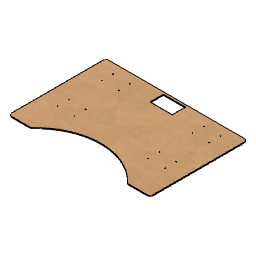
Support_1 (Autodesk Fusion 360 design; units mm, degrees)
Autodesk Fusion 360 part; units mm, degrees
sketch "Esquisse1" plane through (0, 0, 0) normal (0, 1, 0) x (1, 0, 0)
  line L0 (-305, 225) -> (305, 225)
  line L1 (325, 205) -> (325, -205)
  line L2 (305, -225) -> (223.8346, -225)
  line L3 (-325, -205) -> (-325, 205)
  line L4 (-325, 225) -> (325, -225) construction
  line L5 (325, 225) -> (-325, -225) construction
  arc A0 (209.2489, -218.6842) -> (-209.2489, -218.6842) centre (0, -415) ccw
  line L6 (-367.4671, -125) -> (350, -125) construction
  line L7 (-305, -225) -> (-223.8346, -225)
  line L8 (215, -225) -> (325, -225)
  arc A1 (209.2489, -218.6842) -> (223.8346, -225) centre (223.8346, -205) ccw
  arc A2 (305, -225) -> (325, -205) centre (305, -205) ccw
  arc A3 (325, 205) -> (305, 225) centre (305, 205) ccw
  arc A4 (-305, 225) -> (-325, 205) centre (-305, 205) ccw
  arc A5 (-325, -205) -> (-305, -225) centre (-305, -205) ccw
  arc A6 (-223.8346, -225) -> (-209.2489, -218.6842) centre (-223.8346, -205) ccw
  point P0 (-215, -225)
  dimension "d12" = 650
  dimension "d13" = 450
  dimension "d14" = 110
  dimension "d15" = 110
  dimension "d16" = 100
  dimension "d20" = 190
  dimension "d21" = 20
  constraint horizontal L0
  constraint perpendicular L0 L1
  constraint parallel L0 L2
  constraint parallel L1 L3
  constraint coincident L4 origin
  constraint coincident L5 origin
  constraint coincident L2 P0
  constraint perpendicular L1 L6
  constraint perpendicular L1 L8
  constraint tangent A0 A1
  constraint tangent L2 A1
  constraint coincident L4.end L2
  constraint coincident L4.end L1
  constraint tangent L2 A2
  constraint tangent L1 A2
  constraint equal A1 A2
  constraint coincident L5.start L0
  constraint coincident L5.start L1
  constraint tangent L0 A3
  constraint tangent L1 A3
  constraint equal A1 A3
  constraint coincident L4.start L0
  constraint coincident L4.start L3
  constraint tangent L0 A4
  constraint tangent L3 A4
  constraint equal A1 A4
  constraint coincident L5.end L3
  constraint coincident L5.end L7
  constraint tangent L3 A5
  constraint tangent L7 A5
  constraint equal A1 A5
  constraint coincident P0 L7
  constraint coincident P0 A0
  constraint tangent L7 A6
  constraint tangent A0 A6
  constraint equal A1 A6
  measures "d12" distance of L4.start L5.start
  measures "d13" distance of L4.start L5.end
  measures "d14" distance of L3 P0
  measures "d15" distance of L1 L8.start
  measures "d16" distance of L2 L6
  measures "d20" distance of L2 A0.centre
  measures "d21" radius of A1
extrude "Extrusion1" add sketch "Esquisse1" along normal blind 4
sketch "Esquisse2" plane through (0, 4, 0) normal (0, 1, 0) x (-1, 0, 0)
  arc A0 (325, 205) -> (305, 225) centre (305, 205) ccw
  line L0 (305, 225) -> (223.8346, 225)
  arc A1 (223.8346, 225) -> (209.2489, 218.6842) centre (223.8346, 205) ccw
  arc A2 (-209.2489, 218.6842) -> (209.2489, 218.6842) centre (0, 415) ccw
  arc A3 (-209.2489, 218.6842) -> (-223.8346, 225) centre (-223.8346, 205) ccw
  line L1 (-223.8346, 225) -> (-305, 225)
  arc A4 (-305, 225) -> (-325, 205) centre (-305, 205) ccw
  line L2 (-325, 205) -> (-325, -205)
  arc A5 (-325, -205) -> (-305, -225) centre (-305, -205) ccw
  line L3 (-305, -225) -> (305, -225)
  arc A6 (305, -225) -> (325, -205) centre (305, -205) ccw
  line L4 (325, -205) -> (325, 205)
  line L5 (-50, -150) -> (50, -150)
  line L6 (50, -150) -> (50, -210)
  line L7 (50, -210) -> (-50, -210)
  line L8 (50, -210) -> (-50, -150) construction
  line L9 (-50, -210) -> (-50, -150)
  line L10 (-50, -210) -> (50, -150) construction
  point P0 (0, -275)
  point P1 (0, -180)
  dimension "d24" = 60
  dimension "d25" = 100
  dimension "d26" = 15
  constraint horizontal L7
  constraint perpendicular L7 L9
  constraint parallel L5 L7
  constraint parallel L6 L9
  constraint coincident P1 L8
  constraint coincident P1 L10
  measures "d24" distance of L5.start L7.end
  measures "d25" distance of L6 L9
  measures "d26" distance of L3 L7
extrude "Extrusion2" cut sketch "Esquisse2" against normal blind 50 contours L5 L6 L7 L9
sketch "Esquisse3" plane through (0, 4, 0) normal (0, 1, 0) x (-1, 0, 0)
  line L0 (50, -150) -> (50, -210)
  line L1 (50, -210) -> (-50, -210)
  line L2 (-50, -210) -> (-50, -150)
  line L3 (-50, -150) -> (50, -150)
  arc A0 (325, 205) -> (305, 225) centre (305, 205) ccw
  line L4 (305, 225) -> (223.8346, 225)
  arc A1 (223.8346, 225) -> (209.2489, 218.6842) centre (223.8346, 205) ccw
  arc A2 (-209.2489, 218.6842) -> (209.2489, 218.6842) centre (0, 415) ccw
  arc A3 (-209.2489, 218.6842) -> (-223.8346, 225) centre (-223.8346, 205) ccw
  line L5 (-223.8346, 225) -> (-305, 225)
  arc A4 (-305, 225) -> (-325, 205) centre (-305, 205) ccw
  line L6 (-325, 205) -> (-325, -205)
  arc A5 (-325, -205) -> (-305, -225) centre (-305, -205) ccw
  line L7 (-305, -225) -> (305, -225)
  arc A6 (305, -225) -> (325, -205) centre (305, -205) ccw
  line L8 (325, -205) -> (325, 205)
  circle A7 centre (167, 75) radius 2
  circle A8 centre (243, 75) radius 2
  circle A9 centre (243, -175) radius 2
  circle A10 centre (243, -125.0704) radius 2
  circle A11 centre (167, 24.9296) radius 2
  circle A12 centre (243, 24.9296) radius 2
  circle A13 centre (167, -175) radius 2
  circle A14 centre (167, -125.0704) radius 2
  line L9 (205, -263.7962) -> (205, 261.6023) construction
  line L10 (0, -279.9296) -> (0, 210.0704) construction
  circle A15 centre (-243, 75) radius 2
  circle A16 centre (-167, -175) radius 2
  circle A17 centre (-167, -125.0704) radius 2
  circle A18 centre (-243, -125.0704) radius 2
  circle A19 centre (-243, 24.9296) radius 2
  circle A20 centre (-243, -175) radius 2
  circle A21 centre (-167, 75) radius 2
  circle A22 centre (-167, 24.9296) radius 2
  line L11 (-205, -263.7962) -> (-205, 261.6023) construction
  dimension "d29" = 4
  dimension "d30" = 38
  dimension "d31" = 4
  dimension "d32" = 38
  dimension "d33" = 205
  dimension "d34" = 50
  constraint symmetric A9 A13 L9
  constraint symmetric A7 A8 L9
  constraint perpendicular L7 L10
  constraint symmetric L9.end L10 L11.end
  constraint symmetric L9.start L10 L11.start
  constraint symmetric A7 L10 A21
  constraint symmetric A8 L10 A15
  constraint symmetric A9 L10 A20
  constraint symmetric A10 L10 A18
  constraint symmetric A11 L10 A22
  constraint symmetric A12 L10 A19
  constraint symmetric A13 L10 A16
  constraint symmetric A14 L10 A17
  measures "d29" diameter of A9
  measures "d30" distance of A9.centre L9
  measures "d31" diameter of A8
  measures "d32" distance of A8.centre L9
  measures "d33" distance of L9 L10
  measures "d34" distance of L7 A9.centre
extrude "Extrusion3" cut sketch "Esquisse3" against normal blind 25 contours A7 | A8 | A9 | A10 | A11 | A12 | A13 | A14 | A15 | A16 | A17 | A18 | A19 | A20 | A21 | A22
sketch "Esquisse4" plane through (0, 4, 0) normal (0, 1, 0) x (-1, 0, 0)
  circle A0 centre (-243, 24.9296) radius 2
  circle A1 centre (-167, -175) radius 2
  circle A2 centre (167, -175) radius 2
  circle A3 centre (167, 75) radius 2
  circle A4 centre (167, 24.9296) radius 2
  circle A5 centre (243, -125.0704) radius 2
  circle A6 centre (-167, -125.0704) radius 2
  circle A7 centre (-243, 75) radius 2
  circle A8 centre (-167, 24.9296) radius 2
  circle A9 centre (-243, -175) radius 2
  circle A10 centre (243, -175) radius 2
  circle A11 centre (243, 75) radius 2
  circle A12 centre (243, 24.9296) radius 2
  circle A13 centre (167, -125.0704) radius 2
  circle A14 centre (-243, -125.0704) radius 2
  circle A15 centre (-167, 75) radius 2
  line L0 (50, -150) -> (50, -210)
  line L1 (50, -210) -> (-50, -210)
  line L2 (-50, -210) -> (-50, -150)
  line L3 (-50, -150) -> (50, -150)
  arc A16 (325, 205) -> (305, 225) centre (305, 205) ccw
  line L4 (305, 225) -> (223.8346, 225)
  arc A17 (223.8346, 225) -> (209.2489, 218.6842) centre (223.8346, 205) ccw
  arc A18 (-209.2489, 218.6842) -> (209.2489, 218.6842) centre (0, 415) ccw
  arc A19 (-209.2489, 218.6842) -> (-223.8346, 225) centre (-223.8346, 205) ccw
  line L5 (-223.8346, 225) -> (-305, 225)
  arc A20 (-305, 225) -> (-325, 205) centre (-305, 205) ccw
  line L6 (-325, 205) -> (-325, -205)
  arc A21 (-325, -205) -> (-305, -225) centre (-305, -205) ccw
  line L7 (-305, -225) -> (305, -225)
  arc A22 (305, -225) -> (325, -205) centre (305, -205) ccw
  line L8 (325, -205) -> (325, 205)
  line L9 (305, 220) -> (223.8346, 220)
  arc A23 (223.8346, 220) -> (212.8953, 215.2631) centre (223.8346, 205) ccw
  arc A24 (-212.8953, 215.2631) -> (212.8953, 215.2631) centre (0, 415) ccw
  arc A25 (-212.8953, 215.2631) -> (-223.8346, 220) centre (-223.8346, 205) ccw
  line L10 (-223.8346, 220) -> (-305, 220)
  arc A26 (-305, 220) -> (-320, 205) centre (-305, 205) ccw
  line L11 (-320, 205) -> (-320, -205)
  arc A27 (-320, -205) -> (-305, -220) centre (-305, -205) ccw
  line L12 (-305, -220) -> (305, -220)
  arc A28 (305, -220) -> (320, -205) centre (305, -205) ccw
  line L13 (320, -205) -> (320, 205)
  arc A29 (320, 205) -> (305, 220) centre (305, 205) ccw
  dimension "d37" = -5
extrude "Extrusion4" cut sketch "Esquisse4" against normal blind 50 contours A16 L4 A17 A18 A19 L5 A20 L6 A21 L7 A22 L8
